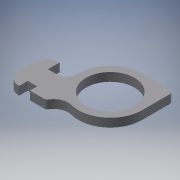
# Autodesk Inventor part: fixed_holder
Saved by Autodesk Inventor 2017.2 (Build 212233000, 233)
## iProperties
Created: 2017-07-16
Part Number: fixed_holder
Material: Generic
Document SubType Name: Modeling
Designer: Nic
Density: 1 g/cm^3
Appearance: Default
Author: Nic
Autodesk Inventor part; units mm, degrees
ref_plane "YZ Plane" through (0, 0, 0) normal (1, 0, 0) x (0, 1, 0)
ref_plane "XZ Plane" through (0, 0, 0) normal (0, 1, 0) x (-1, 0, 0)
ref_plane "XY Plane" through (0, 0, 0) normal (0, 0, 1) x (1, 0, 0)
sketch "Sketch1" plane through (0, 0, 0) normal (0, 0, 1) x (1, 0, 0)
  circle A0 centre (0, 0) radius 16.75
  line L0 (0, 0) -> (-16.1552, 0) construction
  line L1 (-15.7399, -5.7288) -> (0, 0) construction
  line L2 (-14.0236, -9.1597) -> (0, 0) construction
  line L3 (-40, 4.5) -> (-40, -8.5)
  line L4 (-30.5, 14) -> (-30.5, 6)
  line L5 (-30.5, 6) -> (-21.5, 6)
  line L6 (-30.5, -8) -> (-24, -8)
  line L7 (-30.5, -8) -> (-30.5, -18)
  arc A1 (-15.2959, -15.8125) -> (22, 0) centre (0, 0) ccw
  arc A2 (0, 22) -> (-21.0734, 6.3174) centre (0, 0) ccw
  line L8 (-22.2486, -13) -> (-24, -13)
  line L9 (-24, -13) -> (-24, -8)
  line L10 (-40, -2) -> (-34.8901, -2) construction
  arc A3 (-15.2959, -15.8125) -> (-22.2486, -13) centre (-22.2486, -23) ccw
  line L11 (22, 0) -> (22, 19)
  line L12 (0, 22) -> (19, 22)
  arc A4 (22, 19) -> (19, 22) centre (19, 19) ccw
  arc A5 (-40, -8.5) -> (-30.5, -18) centre (-30.5, -8.5) ccw
  arc A6 (-30.5, 14) -> (-40, 4.5) centre (-30.5, 4.5) ccw
  arc A7 (-21.5, 6) -> (-21.0734, 6.3174) centre (-21.5, 6.4453) ccw
  point P0 (-22.2486, -13)
  point P1 (-22, 0)
  dimension "d12" = 16.75
  dimension "d19" = 160
  dimension "d30" = 9
  dimension "d40" = 40
  dimension "d44" = 22
  dimension "d59" = 6.5
  dimension "d61" = 10
  dimension "d68" = 14
  dimension "d69" = 5
  dimension "d71" = 8
  dimension "d73" = 3
  dimension "d78" = 6
  dimension "d79" = 2
  dimension "d80" = 24
  constraints: 26 end point, 23 point on circle, 10 tangent, 8 centre point, 5 horizontal, 4 vertical, 2 coincident, 2 perpendicular, 1 collinear, 1 concentric, 1 horizontal alignment, 1 midpoint, 1 point on line, 1 vertical alignment, 1 other
  measures "d12" radius of A0
  measures "d19" angle of L0 L1
  measures "d30" distance of L4.end L5.end
  measures "d40" distance from line of L3 point (0, 0)
  measures "d44" radius of A2
  measures "d59" distance of L6.start L6.end
  measures "d61" radius of A3
  measures "d68" distance between parallel lines of L5 L6
  measures "d69" distance between parallel lines of L6 L8
  measures "d71" distance of L4.start L4.end
  measures "d73" radius of A4
  measures "d78" distance between parallel lines of L0 L5
  measures "d79" distance between parallel lines of L0 L10
  measures "d80" distance from line of point (0, 0) L9
extrude "Extrusion1" add sketch "Sketch1" along normal blind 5.85
body "Solid1"
